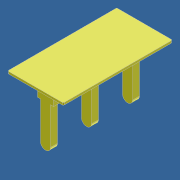
# Autodesk Inventor part: M201203BR-terminals
Saved by Autodesk Inventor 2014 (Build 180170000, 170)
## iProperties
Category: PARTsolutions
Created: 2013-12-29
Part Number: M201203BR-terminals
Catalog Web Link: www.cadenas.de
Description: Bracket Mount Miniature Toggles-terminals - Series M - Miniature Toggles
Document SubType Name: Modeling
Designer: PARTsolutions
Material: Generic
Density: 1 g/cm^3
Appearance: RGB(234,234,0)
NB: M201203BR-terminals
NN: Bracket Mount Miniature Toggles-terminals
NT: Series M - Miniature Toggles
NBSYN: $PN.-terminals
LINA: M201203BR-terminals
PN: M201203BR
SRS: M20
PLS: 1
CRCTSALG: '1','1 - ON/NONE/OFF','2','2 - ON/NONE/ON','3','3 - ON/OFF/ON','5','5 - ON/NONE/(ON)','8','8 - (ON)/OFF/(ON)','9','9 - ON/OFF/(ON)','4', '4 - ON/ON/ON','6','6 - (ON)/ON/(ON)','7','7 - ON/ON/(ON)'
CRCTS: 2
TRMNLSALG: '01','01 - Solder Lug','02','02 - Quick Connect','03','03 - .250" (6.35mm) Straight PC','05', '05 - .425" (10.8mm) Wirewrap','06', '06 - .750" (19.05mm) Wirewrap','07', '07 - .964" (24.5mm) Wirewrap','08', '08 - 1.062" (27.0mm) Wirewrap'
TRMNLS: 03
WIDTH: 0.512
HEIGHT: 0.370
LENGTH: 0.311
A: 0.000
TRMNLNOH: 1.000
POS: 0.000
TRMNLOV: 3.000
KT: DUMMY
SUPPLIER: NKKSWITCHES
ARTICLENO: M201203BR-terminals
BOMINFO: M201203BR-terminals
CREATOR: CADENAS GmbH
PSOL_IDENT_0: {$CADENAS_DATA\23d-libs\nkkswitches\toggle\m\parts\m_br_terminal.prj},231 {VTYP=3D},{NB=M201203BR-te
PSOL_IDENT_1: rminals},{LINA=M201203BR-terminals},{NN=Bracket Mount Miniature Toggles-terminals},{DATE=30.10.2007
PSOL_IDENT_2: 20:08:24},{GEOMDATE=11.05.2007 00:00:00},{VERSION=},{LINEID=10},{LINESUBID=-1},{WBVAR=PLS,CRCTS,TRMN
PSOL_IDENT_3: LS}  {NB=M201203BR-terminals},{LINA=M201203BR-terminals},{KT=DUMMY},{PN=M201203BR},{SRS=M20},{PLS=1}
PSOL_IDENT_4: ,{CRCTSALG='1','1 - ON/NONE/OFF','2','2 - ON/NONE/ON','3','3 - ON/OFF/ON','5','5 - ON/NONE/(ON)','8'
PSOL_IDENT_5: ,'8 - (ON)/OFF/(ON)','9','9 - ON/OFF/(ON)','4', '4 - ON/ON/ON','6','6 - (ON)/ON/(ON)','7','7 - ON/ON
PSOL_IDENT_6: /(ON)'},{CRCTS=2},{TRMNLSALG='01','01 - Solder Lug','02','02 - Quick Connect','03','03 - .250\" (6.3
PSOL_IDENT_7: 5mm) Straight PC','05', '05 - .425\" (10.8mm) Wirewrap','06', '06 - .750\" (19.05mm) Wirewrap','07',
PSOL_IDENT_8: '07 - .964\" (24.5mm) Wirewrap','08', '08 - 1.062\" (27.0mm) Wirewrap'},{TRMNLS=03},{WIDTH=0.512},{
PSOL_IDENT_9: HEIGHT=0.37},{LENGTH=0.311},{A=0},{TRMNLNOH=1},{POS=0},{TRMNLOV=3}
Title: M201203BR-terminals
Author: Cadenas PARTsolutions
Comments: Series M - Miniature Toggles
Autodesk Inventor part; units mm, degrees
sketch "Sketch_2" plane through (0, 0, 0) normal (0, 1, 0) x (-1, 0, 0)
  line L0 (3.1877, -6.1184) -> (3.1877, 6.1184)
  arc A0 (3.1877, 6.1184) -> (3.0577, 6.2484) centre (3.0577, 6.1184) ccw
  line L1 (3.0577, 6.2484) -> (-3.0577, 6.2484)
  arc A1 (-3.0577, 6.2484) -> (-3.1877, 6.1184) centre (-3.0577, 6.1184) ccw
  line L2 (-3.1877, 6.1184) -> (-3.1877, -6.1184)
  arc A2 (-3.1877, -6.1184) -> (-3.0577, -6.2484) centre (-3.0577, -6.1184) ccw
  line L3 (-3.0577, -6.2484) -> (3.0577, -6.2484)
  arc A3 (3.0577, -6.2484) -> (3.1877, -6.1184) centre (3.0577, -6.1184) ccw
  constraints: 8 end point, 8 point on circle, 4 centre point
extrude "Extrusion1" add sketch "Sketch_2" along normal blind 0.254
sketch "Sketch_7" plane through (0, 0, -4.699) normal (0, 0, 1) x (1, 0, 0)
  line L0 (-0.9271, 0) -> (-0.9271, -1.8034)
  line L1 (-0.9271, -1.8034) -> (-0.5842, -1.8034)
  line L2 (-0.5842, -1.8034) -> (-0.5842, -6.0198)
  arc A0 (-0.5842, -6.0198) -> (0.5842, -6.0198) centre (0, -6.0198) ccw
  line L3 (0.5842, -6.0198) -> (0.5842, -1.8034)
  line L4 (0.5842, -1.8034) -> (0.9271, -1.8034)
  line L5 (0.9271, -1.8034) -> (0.9271, 0)
  line L6 (0.9271, 0) -> (-0.9271, 0)
  constraints: 14 end point, 2 point on circle, 1 centre point
extrude "Extrusion2" add sketch "Sketch_7" along normal mid plane 0.7874
pattern_linear "Rectangular Pattern1" count 3 spacing 4.699 along (0, 0, 1) of "Extrusion2"
ref_plane "to_base_XY" through (0, 0, 0) normal (0, 1, 0) x (1, 0, 0)
ref_plane "to_base_YZ" through (0, 0, 0) normal (1, 0, 0) x (0, 0, -1)
ref_plane "to_base_ZX" through (0, 0, 0) normal (0, 0, -1) x (0, 1, 0)
body "Solid1"
